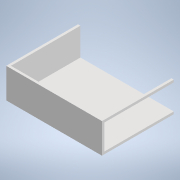
# Autodesk Inventor part: ДИ 00.00.07
Saved by Autodesk Inventor 2021.2 (Build 252289000, 289)
## iProperties
Created: 2021-10-12
Part Number: ДИ 00.00.07
Material: Типовые
Document SubType Name: Modeling
Designer: Surflay
Density: 1 g/cm^3
Appearance: По умолчанию
Author: Surflay
Autodesk Inventor part; units mm, degrees
ref_plane "YZ Plane" through (0, 0, 0) normal (1, 0, 0) x (0, 1, 0)
ref_plane "XZ Plane" through (0, 0, 0) normal (0, 1, 0) x (-1, 0, 0)
ref_plane "XY Plane" through (0, 0, 0) normal (0, 0, 1) x (1, 0, 0)
sketch "Эскиз1" plane through (0, 0, 0) normal (0, 0, 1) x (1, 0, 0)
  line L0 (31.5, 14) -> (-48.5, 14)
  line L1 (-48.5, 14) -> (-48.5, -11)
  line L2 (-48.5, -11) -> (31.5, -11)
  line L3 (31.5, -11) -> (31.5, 14)
  line L4 (33.5, -8.5) -> (33.5, 11.5) projected
  point P0 (0, 0)
  point P1 (31.5, 1.5)
  point P2 (33.5, 1.5)
  dimension "d0" = 80
  dimension "d1" = 25
  dimension "d2" = 2
  constraints: 8 end point, 2 midpoint, 2 parallel, 1 horizontal, 1 horizontal alignment, 1 perpendicular
  measures "d0" distance of L2.end L1.end
  measures "d1" distance of L1.end L0.end
  measures "d2" distance between parallel lines of L4 L3
extrude "Выдавливание1" add sketch "Эскиз1" along normal blind 60
sketch "Эскиз2" plane through (-48.5, 14, 0) normal (0, 1, 0) x (1, 0, 0)
  line L0 (0, 0) -> (80, 0) projected
  line L1 (78, 0) -> (2, 0)
  line L2 (2, 0) -> (2, -58)
  line L3 (2, -58) -> (78, -58)
  line L4 (78, -58) -> (78, 0)
  line L5 (80, -60) -> (0, -60) projected
  line L6 (0, 0) -> (0, -60) projected
  line L7 (80, 0) -> (80, -60) projected
  point P0 (48.5, 0)
  dimension "d5" = 2
  dimension "d6" = 2
  dimension "d7" = 2
  constraints: 8 end point, 2 parallel, 1 horizontal, 1 perpendicular, 1 point on line
  measures "d5" distance between parallel lines of L5 L3
  measures "d6" distance between parallel lines of L6 L2
  measures "d7" distance between parallel lines of L7 L4
extrude "Выдавливание2" cut sketch "Эскиз2" against normal blind 23 contours L0 L4 L3 L2
sketch "Эскиз3" plane through (29.5, 14, 0) normal (-1, 0, 0) x (0, 0, 1)
  line L0 (58, 0) -> (58, -23) projected
  line L1 (0, -23) -> (58, -23) projected
  line L2 (58, -2) -> (0, -2)
  line L3 (0, -2) -> (0, -23)
  line L4 (0, -23) -> (58, -23)
  line L5 (58, -23) -> (58, -2)
  line L6 (0, 0) -> (58, 0) projected
  point P0 (0, -14)
  dimension "d10" = 2
  constraints: 8 end point, 2 parallel, 1 horizontal, 1 perpendicular, 1 point on line
  measures "d10" distance between parallel lines of L6 L2
ref_plane "РабПлоскость1" through (33.5, -8.5, 0) normal (-1, 0, 0) x (0, 0, 1)
extrude "Выдавливание3" cut sketch "Эскиз3" against normal up to surface (4 mm away)
